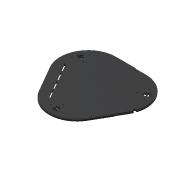
# Autodesk Inventor part: Part6
Saved by Autodesk Inventor 2016 (Build 200138000, 138)
## iProperties
Created: 2016-03-29
Part Number: Part6
Material: ABS Plastic
Document SubType Name: Modeling
Designer: admin
Density: 1 g/cm^3
Appearance: Dark Gray
Author: admin
Autodesk Inventor part; units mm, degrees
ref_plane "YZ Plane" through (0, 0, 0) normal (1, 0, 0) x (0, 1, 0)
ref_plane "XZ Plane" through (0, 0, 0) normal (0, 1, 0) x (-1, 0, 0)
ref_plane "XY Plane" through (0, 0, 0) normal (0, 0, 1) x (1, 0, 0)
sketch "Sketch1" plane through (0, 0, 0) normal (0, 0, 1) x (1, 0, 0)
  circle A0 centre (28, 169.4449) radius 5 projected
  circle A1 centre (188.7436, 229.9186) radius 2 projected
  circle A2 centre (160.7436, 278.416) radius 2 projected
  circle A3 centre (-132.7436, 229.9186) radius 2 projected
  circle A4 centre (-104.7436, 278.416) radius 2 projected
  circle A5 centre (56, 0) radius 2 projected
  circle A6 centre (0, 0) radius 2 projected
  arc A7 (202.3732, 146.7128) -> (95.5, 331.8225) centre (95.5, 208.416) ccw projected
  line L0 (95.5, 331.8225) -> (-39.5, 331.8225) projected
  arc A8 (-39.5, 331.8225) -> (-146.3732, 146.7128) centre (-39.5, 208.416) ccw projected
  line L1 (-146.3732, 146.7128) -> (-78.8732, 29.7993) projected
  arc A9 (-78.8732, 29.7993) -> (134.8732, 29.7993) centre (28, 91.5026) ccw projected
  line L2 (134.8732, 29.7993) -> (202.3732, 146.7128) projected
  arc A10 (-115.4591, 242.4561) -> (-113.4101, 243.0051) centre (-114.7091, 243.7551) ccw projected
  line L3 (-115.4591, 242.4561) -> (-120.1357, 245.1561) projected
  arc A11 (-120.6847, 247.2051) -> (-120.1357, 245.1561) centre (-119.3857, 246.4551) ccw projected
  line L4 (-120.6847, 247.2051) -> (-113.6847, 259.3295) projected
  arc A12 (-111.6357, 259.8785) -> (-113.6847, 259.3295) centre (-112.3857, 258.5795) ccw projected
  line L5 (-111.6357, 259.8785) -> (-106.9591, 257.1785) projected
  arc A13 (-106.4101, 255.1295) -> (-106.9591, 257.1785) centre (-107.7091, 255.8795) ccw projected
  line L6 (-106.4101, 255.1295) -> (-113.4101, 243.0051) projected
  arc A14 (162.9591, 257.1785) -> (162.4101, 255.1295) centre (163.7091, 255.8795) ccw projected
  line L7 (162.9591, 257.1785) -> (167.6357, 259.8785) projected
  arc A15 (169.6847, 259.3295) -> (167.6357, 259.8785) centre (168.3857, 258.5795) ccw projected
  line L8 (169.6847, 259.3295) -> (176.6847, 247.2051) projected
  arc A16 (176.1357, 245.1561) -> (176.6847, 247.2051) centre (175.3857, 246.4551) ccw projected
  line L9 (176.1357, 245.1561) -> (171.4591, 242.4561) projected
  arc A17 (169.4101, 243.0051) -> (171.4591, 242.4561) centre (170.7091, 243.7551) ccw projected
  line L10 (169.4101, 243.0051) -> (162.4101, 255.1295) projected
  arc A18 (36.5, 8.7) -> (35, 10.2) centre (35, 8.7) ccw projected
  line L11 (36.5, 8.7) -> (36.5, 3.3) projected
  arc A19 (35, 1.8) -> (36.5, 3.3) centre (35, 3.3) ccw projected
  line L12 (35, 1.8) -> (21, 1.8) projected
  arc A20 (19.5, 3.3) -> (21, 1.8) centre (21, 3.3) ccw projected
  line L13 (19.5, 3.3) -> (19.5, 8.7) projected
  arc A21 (21, 10.2) -> (19.5, 8.7) centre (21, 8.7) ccw projected
  line L14 (21, 10.2) -> (35, 10.2) projected
  line L15 (-91.8574, 86.3887) -> (-103.8574, 107.1733) projected
  arc A22 (-101.2594, 108.6733) -> (-103.8574, 107.1733) centre (-102.5584, 107.9233) ccw projected
  line L16 (-101.2594, 108.6733) -> (-89.2594, 87.8887) projected
  arc A23 (-91.8574, 86.3887) -> (-89.2594, 87.8887) centre (-90.5584, 87.1387) ccw projected
  circle A24 centre (-62.9327, 116.9449) radius 4.25 projected
  circle A25 centre (28, 274.4449) radius 4.25 projected
  circle A26 centre (118.9327, 116.9449) radius 4.25 projected
  point P0 (0, 0)
extrude "Extrusion1" add sketch "Sketch1" along normal blind 8 contours L2 A9 L1 A8 L0 A7 | L3 A11 L4 A12 L5 A13 L6 A10 | L7 A15 L8 A16 L9 A17 L10 A14 | L11 A19 L12 A20 L13 A21 L14 A18 | L15 A22 L16 A23 | A24 | A25 | A26
sketch "Sketch2" plane through (0, 0, 8) normal (0, 0, 1) x (1, 0, 0)
  circle A0 centre (0, 0) radius 2 projected
  circle A1 centre (56, 0) radius 2 projected
  circle A2 centre (0, 0) radius 12
  circle A3 centre (56, 0) radius 12
  line L0 (0, 12) -> (56, 12)
  line L1 (21, 9.5) -> (35, 9.5)
  line L2 (21, 2.5) -> (35, 2.5)
  line L3 (18, -4.2) -> (18, -7.6)
  line L4 (38, -4.2) -> (38, -7.6)
  line L5 (21, -7.6) -> (35, -7.6)
  line L6 (18, -1.2) -> (38, -1.2)
  line L7 (21, 10.2) -> (35, 10.2)
  line L8 (21, 1.8) -> (35, 1.8)
  line L9 (21, 10.2) -> (21, 1.8)
  line L10 (35, 10.2) -> (35, 1.8)
  arc A4 (18, -1.2) -> (18, -4.2) centre (18, -2.7) ccw
  circle A5 centre (28, 169.4449) radius 5 projected
  circle A6 centre (0, 0) radius 2 projected
  circle A7 centre (56, 0) radius 2 projected
  circle A8 centre (-104.7436, 278.416) radius 2 projected
  circle A9 centre (-132.7436, 229.9186) radius 2 projected
  circle A10 centre (160.7436, 278.416) radius 2 projected
  circle A11 centre (188.7436, 229.9186) radius 2 projected
  arc A12 (202.3732, 146.7128) -> (95.5, 331.8225) centre (95.5, 208.416) ccw projected
  line L11 (95.5, 331.8225) -> (-39.5, 331.8225) projected
  arc A13 (-39.5, 331.8225) -> (-146.3732, 146.7128) centre (-39.5, 208.416) ccw projected
  line L12 (-146.3732, 146.7128) -> (-78.8732, 29.7993) projected
  arc A14 (-78.8732, 29.7993) -> (134.8732, 29.7993) centre (28, 91.5026) ccw projected
  line L13 (134.8732, 29.7993) -> (202.3732, 146.7128) projected
  arc A15 (38, -4.2) -> (38, -1.2) centre (38, -2.7) ccw
  arc A16 (18, -7.6) -> (21, -7.6) centre (19.5, -7.6) ccw
  arc A17 (35, -7.6) -> (38, -7.6) centre (36.5, -7.6) ccw
  arc A18 (21, 10.2) -> (19.5, 8.7) centre (21, 8.7) ccw
  arc A19 (35, 1.8) -> (36.5, 3.3) centre (35, 3.3) ccw
  arc A20 (36.5, 8.7) -> (35, 10.2) centre (35, 8.7) ccw
  line L14 (19.5, 8.7) -> (19.5, 3.3)
  line L15 (36.5, 8.7) -> (36.5, 3.3)
  arc A21 (19.5, 3.3) -> (21, 1.8) centre (21, 3.3) ccw
  dimension "d2" = 24
  dimension "d3" = 24
  dimension "d4" = 2.5
  dimension "d5" = 7
  dimension "d8" = 20
  dimension "d9" = 18
  dimension "d10" = 18
  dimension "d11" = 3.7
  dimension "d12" = 6.4
  dimension "d13" = 0.7
  dimension "d14" = 0.7
  dimension "d15" = 14
  dimension "d16" = 21
  dimension "d17" = 3
  dimension "d18" = 1.5
  dimension "d19" = 1.5
  dimension "d20" = 1.5
  dimension "d21" = 3
  constraints: 26 end point, 16 point on circle, 12 point on line, 9 tangent, 8 centre point, 6 parallel, 4 perpendicular, 2 coincident, 2 horizontal, 2 vertical alignment, 4 other
  measures "d4" distance between parallel lines of L0 L1
  measures "d5" distance between parallel lines of L1 L2
  measures "d8" distance between parallel lines of L4 L3
  measures "d9" distance from line of A0.centre L3
  measures "d10" distance from line of A1.centre L4
  measures "d11" distance between parallel lines of L2 L6
  measures "d12" distance between parallel lines of L6 L5
  measures "d13" distance between parallel lines of L1 L7
  measures "d14" distance between parallel lines of L2 L8
  measures "d15" distance between parallel lines of L10 L9
  measures "d16" distance from line of A0.centre L9
  measures "d17" diameter of A4
  measures "d18" radius of A16
  measures "d19" radius of A17
  measures "d20" radius of A15
  measures "d21" diameter of A18
extrude "Extrusion2" cut sketch "Sketch2" against normal blind 10 contours L9 L7 L10 L1 | L9 A21 L14 A18 | L1 L10 L2 L9 | L10 A20 L15 A19 | L2 L10 L8 L9 | A4 L6 A15 L4 A17 L5 A16 L3
sketch "Sketch3" plane through (0, 0, 8) normal (0, 0, 1) x (1, 0, 0)
  line L0 (19.5, 3.3) -> (19.5, 8.7) projected
  line L1 (18, -1.2) -> (38, -1.2) projected
  line L2 (30, 13.8) -> (30, -1.2)
  line L3 (30, -1.2) -> (26, -1.2)
  line L4 (26, -1.2) -> (26, 13.8)
  arc A0 (30, 13.8) -> (26, 13.8) centre (28, 13.8) ccw
  dimension "d25" = 4
  dimension "d26" = 6.5
  constraints: 6 end point, 2 point on circle, 1 centre point, 1 parallel, 1 point on line
  measures "d25" distance between parallel lines of L2 L4
  measures "d26" distance between parallel lines of L0 L4
extrude "Extrusion3" cut sketch "Sketch3" against normal blind 4
fillet "Fillet1" radius 2 5 edges at (30, 12, 4) (26, 12, 4) (28, 15.8, 4) (30, 0.3, 4) (26, 0.3, 4)
sketch "Sketch4" plane through (0, 0, 8) normal (0, 0, 1) x (1, 0, 0)
  line L0 (35, 1.8) -> (30, 1.8) projected
  line L1 (18, -7.6) -> (18, -4.2) projected
  line L2 (26, 1.8) -> (21, 1.8) projected
  line L3 (22, 1.8) -> (24.5, 1.8)
  line L4 (24.5, 1.8) -> (24.5, -13.2)
  line L5 (24.5, -13.2) -> (22, -13.2)
  line L6 (22, -13.2) -> (22, 1.8)
  line L7 (31.5, 1.8) -> (34, 1.8)
  line L8 (34, 1.8) -> (34, -13.2)
  line L9 (34, -13.2) -> (31.5, -13.2)
  line L10 (31.5, -13.2) -> (31.5, 1.8)
  circle A0 centre (23.25, -13.2) radius 1.25
  circle A1 centre (32.75, -13.2) radius 1.25
  dimension "d31" = 12
  dimension "d32" = 2.5
  dimension "d33" = 2.5
  dimension "d34" = 4
  dimension "d35" = 15
  dimension "d36" = 15
  constraints: 16 end point, 4 parallel, 2 horizontal, 2 horizontal alignment, 2 midpoint, 2 perpendicular, 2 point on line, 4 other
  measures "d31" distance between parallel lines of L6 L8
  measures "d32" distance between parallel lines of L6 L4
  measures "d33" distance between parallel lines of L8 L10
  measures "d34" distance between parallel lines of L1 L6
  measures "d35" distance between parallel lines of L5 L3
  measures "d36" distance between parallel lines of L7 L9
extrude "Extrusion4" cut sketch "Sketch4" against normal blind 2.4
pattern_circular "Circular Pattern1" count 3 over 360 about axis through (28, 169.4449, 0) along (0, 0, 1) of "Fillet1", "Extrusion2", "Extrusion3", "Extrusion4"
sketch "Sketch6" plane through (0, 0, 8) normal (0, 0, 1) x (1, 0, 0)
  arc A0 (202.3732, 146.7128) -> (95.5, 331.8225) centre (95.5, 208.416) ccw projected
  line L0 (95.5, 331.8225) -> (-39.5, 331.8225) projected
  arc A1 (-39.5, 331.8225) -> (-146.3732, 146.7128) centre (-39.5, 208.416) ccw projected
  line L1 (-146.3732, 146.7128) -> (-78.8732, 29.7993) projected
  arc A2 (-78.8732, 29.7993) -> (134.8732, 29.7993) centre (28, 91.5026) ccw projected
  line L2 (134.8732, 29.7993) -> (202.3732, 146.7128) projected
  arc A3 (199.6019, 148.3128) -> (95.5, 328.6225) centre (95.5, 208.416) ccw
  line L3 (199.6019, 148.3128) -> (132.1019, 31.3993)
  arc A4 (-76.1019, 31.3993) -> (132.1019, 31.3993) centre (28, 91.5026) ccw
  line L4 (-76.1019, 31.3993) -> (-143.6019, 148.3128)
  arc A5 (-39.5, 328.6225) -> (-143.6019, 148.3128) centre (-39.5, 208.416) ccw
  line L5 (-39.5, 328.6225) -> (95.5, 328.6225)
  line L6 (168.8487, 95.0466) -> (171.6199, 93.4466)
  dimension "d45" = 3.2
  constraints: 8 end point, 6 point on circle, 3 centre point, 2 point on line, 1 perpendicular, 5 other
  measures "d45" radial gap between concentric circles of A0 A3
extrude "Extrusion6" cut sketch "Sketch6" against normal blind 1
sketch "Sketch7" plane through (0, 0, 8) normal (0, 0, 1) x (1, 0, 0)
  arc A0 (199.6019, 148.3128) -> (95.5, 328.6225) centre (95.5, 208.416) ccw projected
  line L0 (95.5, 328.6225) -> (-39.5, 328.6225) projected
  line L1 (132.1019, 31.3993) -> (199.6019, 148.3128) projected
  line L2 (176.1357, 245.1561) -> (171.4591, 242.4561) projected
  line L3 (162.9591, 257.1785) -> (167.6357, 259.8785) projected
  circle A1 centre (28, 169.4449) radius 5 projected
  line L4 (-39.5, 331.8225) -> (95.5, 331.8225) projected
  line L5 (202.3732, 146.7128) -> (134.8732, 29.7993) projected
  arc A2 (28, 331.8225) -> (168.6232, 88.256) centre (28, 169.4449) ccw
  arc A3 (172.6804, 243.1612) -> (164.1804, 257.8836) centre (28, 169.4449) ccw
  arc A4 (202.3732, 146.7128) -> (95.5, 331.8225) centre (95.5, 208.416) ccw projected
  arc A5 (47.8, 331.8225) -> (51, 328.6225) centre (51, 331.8225) ccw
  arc A6 (177.3519, 109.7746) -> (178.5232, 105.4033) centre (180.1232, 108.1746) ccw
  dimension "d55" = 3.2
  dimension "d56" = 23
  dimension "d57" = 3.2
  dimension "d58" = 23
  constraints: 8 point on circle, 6 point on line, 4 centre point, 2 midpoint, 2 tangent, 1 coincident
  measures "d55" radius of A5
  measures "d56" distance of A2.start A5.centre
  measures "d57" radius of A6
  measures "d58" distance of A2.end A6.centre
extrude "Extrusion7" cut sketch "Sketch7" against normal blind 3 contours A0 L0 A5 L4 A4 L5 A6 L1
sketch "Sketch8" plane through (0, 0, 8) normal (0, 0, 1) x (1, 0, 0)
  arc A0 (-114.7828, 263.4275) -> (-117.3809, 264.9275) centre (-116.0818, 264.1775) ccw projected
  line L0 (-117.3809, 264.9275) -> (-120.3253, 266.6275) projected
  arc A1 (-120.3253, 266.6275) -> (-121.8253, 264.0295) centre (-121.0753, 265.3285) ccw projected
  line L1 (-121.8253, 264.0295) -> (-128.8253, 251.9051) projected
  arc A2 (-128.8253, 251.9051) -> (-130.3253, 249.307) centre (-129.5753, 250.6061) ccw projected
  line L2 (-130.3253, 249.307) -> (-127.3809, 247.607) projected
  arc A3 (-127.3809, 247.607) -> (-124.7828, 246.107) centre (-126.0818, 246.857) ccw projected
  line L3 (-124.7828, 246.107) -> (-114.7828, 263.4275) projected
  arc A4 (-120.6847, 247.2051) -> (-120.1357, 245.1561) centre (-119.3857, 246.4551) ccw projected
  line L4 (-120.1357, 245.1561) -> (-115.4591, 242.4561) projected
  arc A5 (-115.4591, 242.4561) -> (-113.4101, 243.0051) centre (-114.7091, 243.7551) ccw projected
  line L5 (-113.4101, 243.0051) -> (-106.4101, 255.1295) projected
  arc A6 (-106.4101, 255.1295) -> (-106.9591, 257.1785) centre (-107.7091, 255.8795) ccw projected
  line L6 (-106.9591, 257.1785) -> (-111.6357, 259.8785) projected
  arc A7 (-111.6357, 259.8785) -> (-113.6847, 259.3295) centre (-112.3857, 258.5795) ccw projected
  line L7 (-113.6847, 259.3295) -> (-120.6847, 247.2051) projected
  arc A8 (180.7828, 246.107) -> (183.3809, 247.607) centre (182.0818, 246.857) ccw projected
  line L8 (183.3809, 247.607) -> (186.3253, 249.307) projected
  arc A9 (186.3253, 249.307) -> (184.8253, 251.9051) centre (185.5753, 250.6061) ccw projected
  line L9 (184.8253, 251.9051) -> (177.8253, 264.0295) projected
  arc A10 (177.8253, 264.0295) -> (176.3253, 266.6275) centre (177.0753, 265.3285) ccw projected
  line L10 (176.3253, 266.6275) -> (173.3809, 264.9275) projected
  arc A11 (173.3809, 264.9275) -> (170.7828, 263.4275) centre (172.0818, 264.1775) ccw projected
  line L11 (170.7828, 263.4275) -> (180.7828, 246.107) projected
  arc A12 (169.6847, 259.3295) -> (167.6357, 259.8785) centre (168.3857, 258.5795) ccw projected
  line L12 (167.6357, 259.8785) -> (162.9591, 257.1785) projected
  arc A13 (162.9591, 257.1785) -> (162.4101, 255.1295) centre (163.7091, 255.8795) ccw projected
  line L13 (162.4101, 255.1295) -> (169.4101, 243.0051) projected
  arc A14 (169.4101, 243.0051) -> (171.4591, 242.4561) centre (170.7091, 243.7551) ccw projected
  line L14 (171.4591, 242.4561) -> (176.1357, 245.1561) projected
  arc A15 (176.1357, 245.1561) -> (176.6847, 247.2051) centre (175.3857, 246.4551) ccw projected
  line L15 (176.6847, 247.2051) -> (169.6847, 259.3295) projected
  arc A16 (21, 10.2) -> (19.5, 8.7) centre (21, 8.7) ccw projected
  line L16 (19.5, 8.7) -> (19.5, 3.3) projected
  arc A17 (19.5, 3.3) -> (21, 1.8) centre (21, 3.3) ccw projected
  line L17 (21, 1.8) -> (35, 1.8) projected
  arc A18 (35, 1.8) -> (36.5, 3.3) centre (35, 3.3) ccw projected
  line L18 (36.5, 3.3) -> (36.5, 8.7) projected
  arc A19 (36.5, 8.7) -> (35, 10.2) centre (35, 8.7) ccw projected
  line L19 (35, 10.2) -> (21, 10.2) projected
  arc A20 (18, -1.2) -> (18, -4.2) centre (18, -2.7) ccw projected
  line L20 (18, -4.2) -> (18, -7.6) projected
  arc A21 (18, -7.6) -> (21, -7.6) centre (19.5, -7.6) ccw projected
  line L21 (21, -7.6) -> (35, -7.6) projected
  arc A22 (35, -7.6) -> (38, -7.6) centre (36.5, -7.6) ccw projected
  line L22 (38, -7.6) -> (38, -4.2) projected
  arc A23 (38, -4.2) -> (38, -1.2) centre (38, -2.7) ccw projected
  line L23 (38, -1.2) -> (18, -1.2) projected
  circle A24 centre (28, 169.4449) radius 5 projected
  circle A25 centre (0, 0) radius 2 projected
  circle A26 centre (56, 0) radius 2 projected
  circle A27 centre (-104.7436, 278.416) radius 2 projected
  circle A28 centre (-132.7436, 229.9186) radius 2 projected
  circle A29 centre (160.7436, 278.416) radius 2 projected
  circle A30 centre (188.7436, 229.9186) radius 2 projected
  arc A31 (202.3732, 146.7128) -> (95.5, 331.8225) centre (95.5, 208.416) ccw projected
  line L24 (134.8732, 29.7993) -> (202.3732, 146.7128) projected
  arc A32 (-78.8732, 29.7993) -> (134.8732, 29.7993) centre (28, 91.5026) ccw projected
  line L25 (-146.3732, 146.7128) -> (-78.8732, 29.7993) projected
  arc A33 (-39.5, 331.8225) -> (-146.3732, 146.7128) centre (-39.5, 208.416) ccw projected
  line L26 (95.5, 331.8225) -> (-39.5, 331.8225) projected
  arc A34 (201.0741, 147.4628) -> (95.5, 330.3225) centre (95.5, 208.416) ccw
  arc A35 (-77.5741, 30.5493) -> (133.5741, 30.5493) centre (28, 91.5026) ccw
  line L27 (-77.5741, 30.5493) -> (-145.0741, 147.4628)
  arc A36 (-39.5, 330.3225) -> (-145.0741, 147.4628) centre (-39.5, 208.416) ccw
  arc A37 (47.8, 331.8225) -> (51, 328.6225) centre (51, 331.8225) ccw projected
  arc A38 (177.3519, 109.7746) -> (178.5232, 105.4033) centre (180.1232, 108.1746) ccw projected
  arc A39 (48.4019, 331.8225) -> (51.0777, 330.3235) centre (51, 333.3225) ccw
  arc A40 (178.8241, 108.9246) -> (178.8241, 105.9246) centre (181.4222, 107.4246) ccw
  line L28 (-39.5, 330.3225) -> (48.1733, 330.3225)
  line L29 (51, 330.3225) -> (95.5, 330.3225)
  line L30 (201.0741, 147.4628) -> (178.8241, 108.9246)
  line L31 (177.4108, 106.4767) -> (133.5741, 30.5493)
  line L32 (95.5, 328.6225) -> (-39.5, 328.6225) projected
  line L33 (132.1019, 31.3993) -> (199.6019, 148.3128) projected
  line L34 (-115.4591, 242.4561) -> (-120.1357, 245.1561) projected
  line L35 (180.1232, 108.1746) -> (181.8318, 107.1881)
  dimension "d50" = 1.5
  dimension "d51" = 6
  dimension "d52" = 6
  dimension "d59" = 1.7
  dimension "d60" = 0
  dimension "d61" = 0
  constraints: 13 point on circle, 12 end point, 5 centre point, 4 tangent, 3 parallel, 2 point on line, 2 other
  measures "d50" radial gap between concentric circles of A31 A34
  measures "d51" diameter of A39
  measures "d52" diameter of A40
  measures "d59" distance between parallel lines of L32 L29
  measures "d60" horizontal distance of A39.centre A37.centre
  measures "d61" distance from line of A40.centre L35
extrude "Extrusion8" cut sketch "Sketch8" against normal blind 10 contours L24 A40 L30 A34 L29 A39 L26 A31
sketch "Sketch9" plane through (0, 0, 8) normal (0, 0, 1) x (1, 0, 0)
  line L0 (95.5, 328.6225) -> (-39.5, 328.6225) projected
  circle A0 centre (57, 322.8225) radius 1.625
  circle A1 centre (89.5, 322.8225) radius 1.625
  arc A2 (48.4019, 331.8225) -> (51, 330.3225) centre (51, 333.3225) ccw projected
  line L1 (132.1019, 31.3993) -> (199.6019, 148.3128) projected
  line L2 (-115.4591, 242.4561) -> (-120.1357, 245.1561) projected
  circle A3 centre (191.5789, 146.0166) radius 1.625
  circle A4 centre (175.3289, 117.8708) radius 1.625
  line L3 (199.6019, 148.3128) -> (198.5484, 148.921)
  dimension "d62" = 3.25
  dimension "d63" = 3.25
  dimension "d64" = 5.8
  dimension "d65" = 5.8
  dimension "d66" = 6
  dimension "d67" = 6
  dimension "d70" = 3.25
  dimension "d71" = 3.25
  dimension "d72" = 5.8
  dimension "d73" = 5.8
  dimension "d74" = 6
  dimension "d75" = 32.5
  constraints: 4 centre point, 2 end point, 1 parallel
  measures "d62" diameter of A0
  measures "d63" diameter of A1
  measures "d64" distance from line of L0 A0.centre
  measures "d65" distance from line of L0 A1.centre
  measures "d66" horizontal distance of A0.centre A2.centre
  measures "d67" horizontal distance of L0.start A1.centre
  measures "d70" diameter of A3
  measures "d71" diameter of A4
  measures "d72" distance from line of L1 A4.centre
  measures "d73" distance from line of L1 A3.centre
  measures "d74" distance from line of L3 A3.centre
  measures "d75" distance of A3.centre A4.centre
extrude "Extrusion9" cut sketch "Sketch9" against normal blind 15
thread "Thread1" size "M3.5x0.6" class "6H" standard "ANSI Metric M Profile" full length
thread "Thread2" size "M3.5x0.6" class "6H" standard "ANSI Metric M Profile" full length
thread "Thread3" size "M3.5x0.6" class "6H" standard "ANSI Metric M Profile" full length
thread "Thread4" size "M3.5x0.6" class "6H" standard "ANSI Metric M Profile" full length
sketch "Sketch11" plane through (0, 0, 5) normal (0, 0, 1) x (1, 0, 0)
  arc A0 (201.0741, 147.4628) -> (95.5, 330.3225) centre (95.5, 208.416) ccw projected
  circle A1 centre (210.3217, 167.4628) radius 5
  point P0 (0, 0)
  dimension "d87" = 10
  dimension "d88" = 20
  constraints: 1 centre point, 1 point on circle
  measures "d87" diameter of A1
  measures "d88" vertical distance of A0.start A1.centre
extrude "Extrusion11" cut sketch "Sketch11" along normal mid plane 20
sketch "Sketch12" plane through (0, 0, 8) normal (0, 0, 1) x (1, 0, 0)
  circle A0 centre (28, 169.4449) radius 5 projected
  line L0 (95.5, 328.6225) -> (-39.5, 328.6225) projected
  line L1 (-92, 238.7269) -> (148, 238.7269)
  line L2 (148, 238.7269) -> (28, 30.8808)
  line L3 (28, 30.8808) -> (-92, 238.7269)
  circle A1 centre (-92, 238.7269) radius 3.75
  circle A2 centre (148, 238.7269) radius 3.75
  circle A3 centre (28, 30.8808) radius 3.75
  dimension "d91" = 240
  dimension "d92" = 7.5
  dimension "d93" = 7.5
  dimension "d94" = 7.5
  constraints: 6 end point, 4 coincident, 3 centre point, 1 parallel, 7 other
  measures "d91" distance of L1.start L1.end
  measures "d92" diameter of A1
  measures "d93" diameter of A2
  measures "d94" diameter of A3
extrude "Extrusion12" cut sketch "Sketch12" against normal blind 2 contours L3 A1 L1 | L1 A1 L3 | A2 L2 L1 | L1 L2 A2 | A3 L2 L3 | L3 L2 A3
hole "Hole1" at (-92, 238.7269, 6) direction (0, 0, -1) diameter 3 end through all
hole "Hole2" at (28, 30.8808, 6) direction (0, 0, -1) diameter 3 end through all
hole "Hole3" at (148, 238.7269, 6) direction (0, 0, -1) diameter 3 end through all
sketch "Sketch14" plane through (0, 0, 8) normal (0, 0, 1) x (1, 0, 0)
  circle A0 centre (165.5, 183.416) radius 6 projected
  circle A1 centre (148.5, 297.416) radius 9 projected
  arc A2 (92.906, 305.575) -> (87.5815, 292.3963) centre (91.0739, 298.6502) ccw projected
  line L0 (92.906, 305.575) -> (112.0891, 300.4997) projected
  arc A3 (104.9063, 282.7215) -> (112.0891, 300.4997) centre (109.6176, 291.1581) ccw projected
  line L1 (104.9063, 282.7215) -> (87.5815, 292.3963) projected
  circle A4 centre (7.5591, 129.2849) radius 1.5 projected
  circle A5 centre (169.4725, 139.7272) radius 1.5 projected
  circle A6 centre (124.4725, 61.7849) radius 1.5 projected
  circle A7 centre (52.5591, 207.2272) radius 1.5 projected
  circle A8 centre (191.5789, 146.0166) radius 1.65 projected
  circle A9 centre (89.5, 322.8225) radius 1.65 projected
  circle A10 centre (57, 322.8225) radius 1.65 projected
  circle A11 centre (175.3289, 117.8708) radius 1.65 projected
  arc A12 (207.563, 162.7047) -> (208.3577, 162.3254) centre (210.3217, 167.4628) ccw projected
  line L2 (207.563, 162.7047) -> (202.8842, 165.4175) projected
  arc A13 (205.8573, 173.7531) -> (202.8842, 165.4175) centre (205.1414, 169.3104) ccw projected
  line L3 (205.8573, 173.7531) -> (211.1967, 172.8927) projected
  arc A14 (212.0521, 172.6835) -> (211.1967, 172.8927) centre (210.3217, 167.4628) ccw projected
  arc A15 (212.0521, 172.6835) -> (95.5, 330.3225) centre (95.5, 208.416) ccw projected
  line L4 (95.5, 330.3225) -> (51, 330.3225) projected
  arc A16 (48.4019, 331.8225) -> (51, 330.3225) centre (51, 333.3225) ccw projected
  line L5 (48.4019, 331.8225) -> (-39.5, 331.8225) projected
  arc A17 (-39.5, 331.8225) -> (-146.3732, 146.7128) centre (-39.5, 208.416) ccw projected
  line L6 (-146.3732, 146.7128) -> (-78.8732, 29.7993) projected
  arc A18 (-78.8732, 29.7993) -> (134.8732, 29.7993) centre (28, 91.5026) ccw projected
  line L7 (134.8732, 29.7993) -> (178.8241, 105.9246) projected
  arc A19 (178.8241, 108.9246) -> (178.8241, 105.9246) centre (181.4222, 107.4246) ccw projected
  line L8 (178.8241, 108.9246) -> (201.0741, 147.4628) projected
  arc A20 (201.0741, 147.4628) -> (208.3577, 162.3254) centre (95.5, 208.416) ccw projected
  circle A21 centre (0, 0) radius 2 projected
  circle A22 centre (56, 0) radius 2 projected
  circle A23 centre (-104.7436, 278.416) radius 2 projected
  circle A24 centre (-132.7436, 229.9186) radius 2 projected
  circle A25 centre (160.7436, 278.416) radius 2 projected
  circle A26 centre (188.7436, 229.9186) radius 2 projected
  circle A27 centre (28, 169.4449) radius 5 projected
  arc A28 (36.5, 8.7) -> (35, 10.2) centre (35, 8.7) ccw projected
  line L9 (36.5, 8.7) -> (36.5, 3.3) projected
  arc A29 (35, 1.8) -> (36.5, 3.3) centre (35, 3.3) ccw projected
  line L10 (35, 1.8) -> (21, 1.8) projected
  arc A30 (19.5, 3.3) -> (21, 1.8) centre (21, 3.3) ccw projected
  line L11 (19.5, 3.3) -> (19.5, 8.7) projected
  arc A31 (21, 10.2) -> (19.5, 8.7) centre (21, 8.7) ccw projected
  line L12 (21, 10.2) -> (35, 10.2) projected
  arc A32 (162.9591, 257.1785) -> (162.4101, 255.1295) centre (163.7091, 255.8795) ccw projected
  line L13 (162.9591, 257.1785) -> (167.6357, 259.8785) projected
  arc A33 (169.6847, 259.3295) -> (167.6357, 259.8785) centre (168.3857, 258.5795) ccw projected
  line L14 (169.6847, 259.3295) -> (176.6847, 247.2051) projected
  arc A34 (176.1357, 245.1561) -> (176.6847, 247.2051) centre (175.3857, 246.4551) ccw projected
  line L15 (176.1357, 245.1561) -> (171.4591, 242.4561) projected
  arc A35 (169.4101, 243.0051) -> (171.4591, 242.4561) centre (170.7091, 243.7551) ccw projected
  line L16 (169.4101, 243.0051) -> (162.4101, 255.1295) projected
  arc A36 (-115.4591, 242.4561) -> (-113.4101, 243.0051) centre (-114.7091, 243.7551) ccw projected
  line L17 (-115.4591, 242.4561) -> (-120.1357, 245.1561) projected
  arc A37 (-120.6847, 247.2051) -> (-120.1357, 245.1561) centre (-119.3857, 246.4551) ccw projected
  line L18 (-120.6847, 247.2051) -> (-113.6847, 259.3295) projected
  arc A38 (-111.6357, 259.8785) -> (-113.6847, 259.3295) centre (-112.3857, 258.5795) ccw projected
  line L19 (-111.6357, 259.8785) -> (-106.9591, 257.1785) projected
  arc A39 (-106.4101, 255.1295) -> (-106.9591, 257.1785) centre (-107.7091, 255.8795) ccw projected
  line L20 (-106.4101, 255.1295) -> (-113.4101, 243.0051) projected
  arc A40 (-101.1295, 108.7483) -> (-104.1606, 106.9983) centre (-102.645, 107.8733) ccw projected
  line L21 (-101.1295, 108.7483) -> (-89.1295, 87.9637) projected
  arc A41 (-92.1606, 86.2137) -> (-89.1295, 87.9637) centre (-90.645, 87.0887) ccw projected
  line L22 (-92.1606, 86.2137) -> (-104.1606, 106.9983) projected
  circle A42 centre (123.2628, 114.4449) radius 4.25 projected
  circle A43 centre (-67.2628, 114.4449) radius 4.25 projected
  circle A44 centre (28, 279.4449) radius 4.25 projected
  arc A45 (208.3577, 162.3254) -> (212.0521, 172.6835) centre (211.8017, 166.9349) ccw
  constraints: 2 point on circle, 1 centre point
extrude "Extrusion14" cut sketch "Sketch14" against normal blind 10 contours L2 A13 L3 A14 A45 A12
sketch "Sketch16" plane through (0, 0, 8) normal (0, 0, 1) x (1, 0, 0)
  line L0 (-127.0753, 254.9362) -> (-123.5753, 260.9984) projected
  circle A0 centre (-129.6555, 260.4673) radius 1.5
  dimension "d146" = 3
  dimension "d147" = 5
  constraints: 1 centre point
  measures "d146" diameter of A0
  measures "d147" distance from line of L0 A0.centre
hole "Hole4" at (-129.6555, 260.4673, 8) direction (0, 0, -1) diameter 2.459 depth 7 tip angle 118 thread size "M3x0.5" class "6H" standard "ISO Metric profile"
pattern_circular "Circular Pattern2" count 3 over 360 about axis through (28, 169.4449, 0) along (0, 0, 1) of "Hole4"
sketch "Sketch17" plane through (0, 0, 8) normal (0, 0, 1) x (1, 0, 0)
  line L0 (-143.6019, 148.3128) -> (-76.1019, 31.3993) projected
  line L1 (162.9591, 257.1785) -> (167.6357, 259.8785) projected
  line L2 (-127.041, 189.6284) -> (-32.041, 25.0836)
  line L3 (-32.041, 25.0836) -> (-26.8449, 28.0836)
  line L4 (-26.8449, 28.0836) -> (-121.8449, 192.6284)
  line L5 (-121.8449, 192.6284) -> (-127.041, 189.6284)
  line L6 (-101.5949, 157.5544) -> (-106.791, 154.5544)
  line L7 (-96.8449, 149.3272) -> (-102.041, 146.3272)
  line L8 (-76.5949, 114.2532) -> (-81.791, 111.2532)
  line L9 (-72.0949, 106.4589) -> (-77.291, 103.4589)
  line L10 (-51.8449, 71.3849) -> (-57.041, 68.3849)
  line L11 (-47.0949, 63.1577) -> (-52.291, 60.1577)
  line L12 (-79.541, 107.356) -> (-109.8519, 89.856)
  dimension "d162" = 6
  dimension "d163" = 190
  dimension "d164" = 9.5
  dimension "d165" = 9
  dimension "d166" = 9.5
  dimension "d167" = 40.5
  dimension "d168" = 40.5
  dimension "d169" = 40.5
  dimension "d170" = 35
  constraints: 20 end point, 6 point on line, 2 parallel, 1 midpoint, 19 other
  measures "d163" distance between parallel lines of L5 L3
  measures "d164" distance between parallel lines of L7 L6
  measures "d165" distance between parallel lines of L9 L8
  measures "d166" distance between parallel lines of L10 L11
  measures "d167" distance between parallel lines of L5 L6
  measures "d168" distance between parallel lines of L7 L8
  measures "d169" distance between parallel lines of L3 L11
extrude "Extrusion15" cut sketch "Sketch17" against normal blind 10 contours L5 L4 L6 L2 | L7 L4 L8 L2 | L9 L4 L10 L2 | L11 L4 L3 L2
fillet "Fillet2" radius 2 16 edges at (-101.5949, 157.5544, 4) (-106.791, 154.5544, 4) (-127.041, 189.6284, 4) (-121.8449, 192.6284, 4) (-102.041, 146.3272, 4) (-96.8449, 149.3272, 4) (-81.791, 111.2532, 4) (-76.5949, 114.2532, 4) (-77.291, 103.4589, 4) (-72.0949, 106.4589, 4) (-57.041, 68.3849, 4) (-51.8449, 71.3849, 4) (-52.291, 60.1577, 4) (-47.0949, 63.1577, 4) (-32.041, 25.0836, 4) (-26.8449, 28.0836, 4)
sketch "Sketch18" plane through (0, 0, 0) normal (0, 0, -1) x (-1, 0, 0)
  circle A0 centre (-28, 169.4449) radius 5 projected
extrude "Extrusion16" add sketch "Sketch18" against normal blind 8
body "Solid1"
